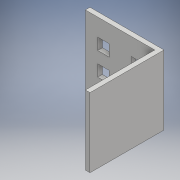
# Autodesk Inventor part: Head
Saved by Autodesk Inventor 2018 (Build 220112000, 112)
## iProperties
Created: 2018-04-26
Part Number: Head
Material: Generic
Document SubType Name: Modeling
Designer: HP
Density: 1 g/cm^3
Appearance: Default
Author: HP
Autodesk Inventor part; units mm, degrees
ref_plane "YZ Plane" through (0, 0, 0) normal (1, 0, 0) x (0, 1, 0)
ref_plane "XZ Plane" through (0, 0, 0) normal (0, 1, 0) x (-1, 0, 0)
ref_plane "XY Plane" through (0, 0, 0) normal (0, 0, 1) x (1, 0, 0)
sketch "Sketch1" plane through (0, 0, 0) normal (0, 1, 0) x (-1, 0, 0)
  line L0 (0, 0) -> (30, 0)
  line L1 (30, 0) -> (30, -30)
  line L2 (30, -30) -> (0, -30)
  line L3 (0, -30) -> (0, 0)
  dimension "d0" = 30
  dimension "d1" = 30
  constraints: 8 end point, 2 parallel, 1 horizontal, 1 perpendicular
  measures "d0" distance of L1.end L2.end
  measures "d1" distance of L0.end L1.end
extrude "Extrusion1" add sketch "Sketch1" along normal blind 2
sketch "Sketch2" plane through (0, 2, 0) normal (0, 1, 0) x (1, 0, 0)
  line L0 (-24.6588, 7.5) -> (-19.6588, 7.5)
  line L1 (-19.6588, 7.5) -> (-19.6588, 12.5)
  line L2 (-19.6588, 12.5) -> (-24.6588, 12.5)
  line L3 (-24.6588, 12.5) -> (-24.6588, 7.5)
  line L4 (-30, 0) -> (0, 0) projected
  line L5 (-24.6588, 17.5) -> (-19.6588, 17.5)
  line L6 (-19.6588, 17.5) -> (-19.6588, 22.5)
  line L7 (-19.6588, 22.5) -> (-24.6588, 22.5)
  line L8 (-24.6588, 22.5) -> (-24.6588, 17.5)
  line L9 (-10.1588, 7.5) -> (-5.1588, 7.5)
  line L10 (-5.1588, 7.5) -> (-5.1588, 22.5)
  line L11 (-5.1588, 22.5) -> (-10.1588, 22.5)
  line L12 (-10.1588, 22.5) -> (-10.1588, 7.5)
  dimension "d4" = 5
  dimension "d5" = 5
  dimension "d6" = 7.5
  dimension "d7" = 5
  dimension "d8" = 5
  dimension "d9" = 5
  dimension "d10" = 9.5
  constraints: 24 end point, 6 parallel, 3 horizontal, 3 perpendicular
  measures "d4" distance of L2.end L1.end
  measures "d5" distance of L1.end L0.end
  measures "d6" distance between parallel lines of L4 L0
  measures "d7" distance of L6.end L5.end
  measures "d8" distance between parallel lines of L5 L2
  measures "d9" distance of L11.end L10.end
  measures "d10" distance between parallel lines of L12 L1
extrude "Extrusion2" cut sketch "Sketch2" against normal blind 2
sketch "Sketch3" plane through (0, 0, 0) normal (1, 0, 0) x (0, 0, -1)
  line L0 (30, 2) -> (0, 2) projected
  line L1 (30, 2) -> (0, 2)
  line L2 (0, 2) -> (0, -30)
  line L3 (0, -30) -> (30, -30)
  line L4 (30, -30) -> (30, 2)
  dimension "d15" = 32
  constraints: 8 end point, 2 parallel, 1 horizontal, 1 perpendicular
  measures "d15" distance of L2.end L1.end
extrude "Extrusion3" add sketch "Sketch3" along normal blind 2
body "Solid1"
